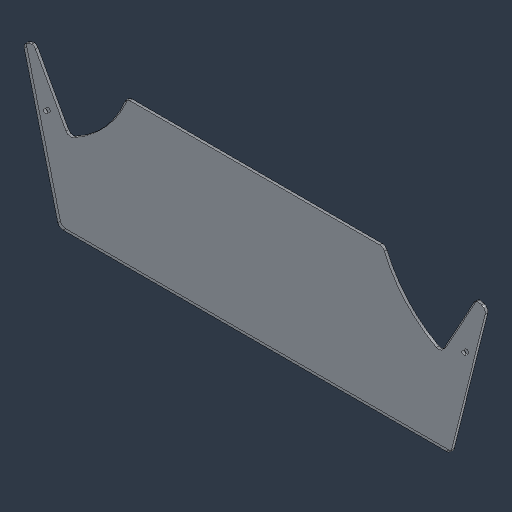
# Autodesk Inventor part: hopper_backboard
Saved by Autodesk Inventor 2024.3 (Build 283343000, 343)
## iProperties
Created: 2025-03-06
Part Number: hopper_backboard
Material: Polycarbonate, Clear
Document SubType Name: Sheet Metal
Designer: marcu
Density: 1.2 g/cm^3
Sheet Metal Rule: Default
Appearance: Polycarbonate - Clear
Mass: 299.19 g
Surface Area: 1683.99 cm^2
Volume: 249.325 cm^3
Author: marcu
Autodesk Inventor part; units mm, degrees
ref_plane "YZ Plane" through (0, 0, 0) normal (1, 0, 0) x (0, 1, 0)
ref_plane "XZ Plane" through (0, 0, 0) normal (0, 1, 0) x (-1, 0, 0)
ref_plane "XY Plane" through (0, 0, 0) normal (0, 0, 1) x (1, 0, 0)
sketch "Sketch1" plane through (0, 0, 0) normal (0, 0, 1) x (1, 0, 0)
  line L0 (185.5464, -240.4953) -> (305.904, 241.6889) construction
  line L1 (192.2769, 35.1785) -> (305.904, 241.6889) construction
  line L2 (288.9878, 173.9183) -> (271.0751, 178.3894)
  line L3 (271.0751, 178.3894) -> (0, 178.3894)
  line L4 (0, 0) -> (0, 127) construction
  line L5 (288.9878, 173.9183) -> (242.8528, -10.9109)
  line L6 (242.8528, -10.9109) -> (0, -10.9109)
  line L7 (-288.9878, 173.9183) -> (-271.0751, 178.3894)
  line L8 (-271.0751, 178.3894) -> (0, 178.3894)
  line L9 (-288.9878, 173.9183) -> (-242.8528, -10.9109)
  line L10 (-242.8528, -10.9109) -> (0, -10.9109)
  line L11 (0, -4.5609) -> (237.893, -4.5609)
  line L12 (237.893, -4.5609) -> (281.289, 169.2951)
  line L13 (281.289, 169.2951) -> (270.2945, 172.0394)
  line L14 (270.2945, 172.0394) -> (0, 172.0394)
  line L15 (0, 172.0394) -> (-270.2945, 172.0394)
  line L16 (-270.2945, 172.0394) -> (-281.289, 169.2951)
  line L17 (-281.289, 169.2951) -> (-237.893, -4.5609)
  line L18 (-237.893, -4.5609) -> (0, -4.5609)
  dimension "d0" = 69.85
  dimension "d1" = 127
  dimension "d2" = 190.5
  dimension "d4" = 6.35
  measures "d0" distance from line of L0.end L2
  measures "d1" distance of L4.start L4.end
  measures "d2" distance of L2.start L5.end
  measures "d4" distance between parallel lines of L6 L11
extrude "Plate1" add sketch "Sketch1" along normal blind 3.048 contours L18 L17 L16 L15 L14 L13 L12 L11
fillet "Corner Round1" radius 6.35 4 edges at (237.893, -4.5609, 1.524) (-237.893, -4.5609, 1.524) (-281.289, 169.2951, 1.524) (281.289, 169.2951, 1.524)
sketch "Sketch6" plane through (0, 0, 3.048) normal (0, 0, 1) x (1, 0, 0)
  line L0 (232.9332, -4.5609) -> (-232.9332, -4.5609) construction
  line L1 (0, -4.5609) -> (0, 109.7391)
  point P0 (0, 0)
  point P1 (254, 109.7391)
  point P2 (-254, 109.7391)
  dimension "d22" = 114.3
  dimension "d23" = 254
  dimension "d24" = 254
  constraints: 2 end point, 2 horizontal alignment, 1 midpoint, 1 vertical
  measures "d22" distance of L1.start L1.end
  measures "d23" distance of point (254, 109.739) L1.end
  measures "d24" distance of point (-254, 109.739) L1.end
hole "Hole1" at (254, 109.7391, 3.048) at (-254, 109.7391, 3.048) direction (0, 0, -1) diameter 5.1054 end through all clearance for "Flat Head Machine Screw (82)" size "#10" standard "Ansi Unified Screw Threads"
sketch "Sketch7" plane through (0, 0, 3.048) normal (0, 0, 1) x (1, 0, 0)
  circle A0 centre (-254, 109.7391) radius 2.5527 construction
  circle A1 centre (254, 109.7391) radius 2.5527 construction
  arc A2 (279.7512, 163.1341) -> (275.128, 170.8329) centre (273.5902, 164.672) ccw construction
  line L0 (270.2945, 172.0394) -> (275.128, 170.8329) construction
  line L1 (-270.2945, 172.0394) -> (270.2945, 172.0394) projected
  line L2 (-275.128, 170.8329) -> (-270.2945, 172.0394) construction
  arc A3 (-275.128, 170.8329) -> (-279.7512, 163.1341) centre (-273.5902, 164.672) ccw construction
  line L3 (-239.0941, 0.2513) -> (-279.7512, 163.1341) construction
  arc A4 (-239.0941, 0.2513) -> (-232.9332, -4.5609) centre (-232.9332, 1.7891) ccw construction
  line L4 (232.9332, -4.5609) -> (-232.9332, -4.5609) construction
  arc A5 (232.9332, -4.5609) -> (239.0941, 0.2513) centre (232.9332, 1.7891) ccw construction
  line L5 (279.7512, 163.1341) -> (239.0941, 0.2513) construction
  line L6 (192.2769, 34.45) -> (305.904, 240.9604)
  arc A6 (155.9945, 172.0394) -> (226.0549, 95.8394) centre (286.5455, 221.7639) ccw
  line L7 (0, 172.0394) -> (0, 146.6394) construction
  line L8 (-192.2769, 34.45) -> (-305.904, 240.9604)
  arc A7 (-226.0549, 95.8394) -> (-155.9945, 172.0394) centre (-286.5455, 221.7639) ccw
  line L9 (267.982, 172.0394) -> (-267.982, 172.0394)
  line L10 (-267.982, 172.0394) -> (-155.9945, 172.0394)
  point P0 (0, 0)
  dimension "d32" = 139.7
  dimension "d33" = 76.2
  dimension "d34" = 114.3
  dimension "d35" = 25.4
  constraints: 10 end point, 7 point on line, 5 symmetric about line, 4 point on circle, 2 centre point, 1 collinear, 1 midpoint, 1 vertical, 4 other
  measures "d32" radius of A6
  measures "d33" distance from line of L1 A6.end
  measures "d34" distance of L0.start A6.start
  measures "d35" distance of L7.start L7.end
extrude "Cut3" cut sketch "Sketch7" against normal blind 3.048
fillet "Corner Round2" radius 6.35 6 edges at (226.0549, 95.8394, 1.524) (155.9945, 172.0394, 1.524) (267.982, 172.0394, 1.524) (-155.9945, 172.0394, 1.524) (-226.0549, 95.8394, 1.524) (-267.982, 172.0394, 1.524)
equation "\"d30\" = Thickness"
equation "\"d36\" = Thickness"
equation "\"d3\" = Thickness"
equation "\"BendRadius\" = Thickness"
equation "\"BendReliefWidth\" = Thickness"
equation "\"BendReliefDepth\" = 0.5 * Thickness"
equation "\"CornerReliefSize\" = 4 * Thickness"
equation "\"MinimumRemnant\" = 2 * Thickness"
equation "\"TransitionRadius\" = BendRadius"
equation "\"JacobiRadiusSize\" = BendRadius"
equation "\"GapSize\" = Thickness"
equation "\"Thickness\" = 3.048"
body "Solid1"
